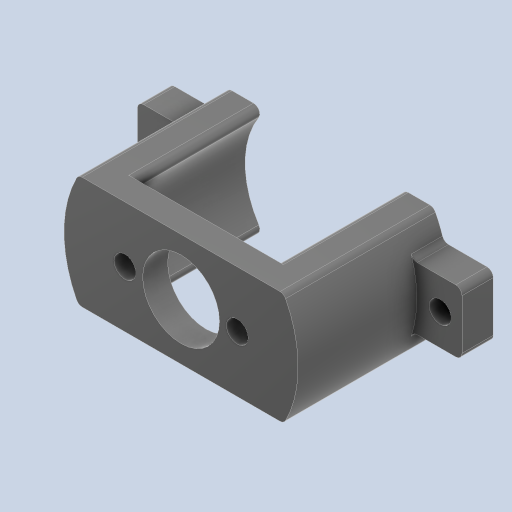
# Autodesk Inventor part: encoderholder
Saved by Autodesk Inventor 2024 (Build 280153000, 153)
## iProperties
Created: 2023-08-25
Part Number: encoderholder
Material: ABS プラスチック
Document SubType Name: Modeling
Designer: zegi
Density: 1.06 g/cm^3
Appearance: 滑らか - 黒
Author: zegi
Autodesk Inventor part; units mm, degrees
ref_plane "YZ Plane" through (0, 0, 0) normal (1, 0, 0) x (0, 1, 0)
ref_plane "XZ Plane" through (0, 0, 0) normal (0, 1, 0) x (-1, 0, 0)
ref_plane "XY Plane" through (0, 0, 0) normal (0, 0, 1) x (1, 0, 0)
sketch "スケッチ2" plane through (0, 0, 0) normal (0, 0, 1) x (1, 0, 0)
  circle A0 centre (0, 0) radius 6.15
  circle A1 centre (9, 0) radius 1.75
  line L0 (0, 9) -> (16.4488, 9)
  line L1 (16.4488, -9) -> (0, -9)
  line L2 (0, -9) -> (0, 9)
  line L3 (0, 0) -> (10.75, 0) construction
  circle A2 centre (0, 0) radius 18.75
  line L4 (0, 0) -> (18.75, 0) construction
  circle A3 centre (0, 0) radius 13.75
  line L5 (0, 0) -> (13.75, 0)
  point P0 (0, 6.15)
  point P1 (0, -6.15)
  point P2 (10.3953, 9)
  point P3 (10.3953, -9)
  dimension "d6" = 3.5
  dimension "d5" = 12.3
  dimension "d7" = 9
  dimension "d11" = 18
  dimension "d12" = 5
  dimension "d20" = 3
  constraints: 12 end point, 3 coincident, 3 point on circle, 2 centre point, 2 horizontal, 2 horizontal alignment, 1 midpoint, 1 parallel, 1 perpendicular, 1 point on line, 1 vertical, 5 other
  measures "d5" diameter of A0
  measures "d7" distance of point (0, 0) point (9, 0)
  measures "d11" distance of L1.end L0.start
  measures "d20" distance of L5.end L3.end
extrude "押し出し1" add sketch "スケッチ2" along normal blind 4 contours L5 A1 A3 L1 L2 A0 | A0 L2 L0 A3 L5 A1 | L0 A2 L1 A3 picked at (14.4338, 5.2266)
extrude "押し出し2" add sketch "スケッチ2" against normal blind 15 contours L0 A2 L1 A3 picked at (14.4338, 5.2266)
sketch "スケッチ3" plane through (0, 0, -15) normal (0, 0, -1) x (-1, 0, 0)
  line L0 (-16.4488, -9) -> (-10.3953, -9) projected
  arc A0 (-10.3953, 9) -> (-10.3953, -9) centre (0, 0) ccw projected
  line L1 (-10.3953, 9) -> (-16.4488, 9) projected
  arc A1 (-16.4488, 9) -> (-16.4488, -9) centre (0, 0) ccw projected
  line L2 (-26, -9) -> (-10.3953, -9)
  line L3 (-10.3953, -9) -> (-10.3953, 9)
  line L4 (-10.3953, 9) -> (-26, 9)
  line L5 (-26, 9) -> (-26, -9)
  line L6 (-26, 0) -> (-10.3953, 0) construction
  circle A2 centre (-22.5, 0) radius 1.75
  line L7 (-26, 5) -> (-10.3953, 5)
  line L8 (-10.3953, 5) -> (-10.3953, -5)
  line L9 (-10.3953, -5) -> (-26, -5)
  line L10 (-26, -5) -> (-26, 5)
  point P0 (-18.071, -5)
  point P1 (-18.071, 5)
  point P2 (-26, -5)
  dimension "d17" = 3.5
  dimension "d18" = 22.5
  dimension "d19" = 3.5
  dimension "d24" = 10
  constraints: 18 end point, 4 parallel, 3 point on line, 2 horizontal, 2 midpoint, 2 perpendicular, 1 centre point, 1 other
  measures "d17" diameter of A2
  measures "d18" distance of A2.centre point (0, 0)
  measures "d19" distance from line of L5 A2.centre
  measures "d24" distance of L7.end L8.end
extrude "押し出し3" add sketch "スケッチ3" along normal blind 5 contours A1 L9 A0 L0 | L9 L5 L7 A1 | A1 L7 A0 L9 | A1 L1 A0 L7
fillet "フィレット1" radius 1 10 edges at (10.3953, 9, -10) (10.3953, -9, -10) (16.4488, 9, -5.5) (16.4488, 9, -17.5) (16.4488, -9, -17.5) (16.4488, -9, -5.5) (26, 5, -17.5) (26, -5, -17.5) (18.071, 5, -17.5) (18.071, -5, -17.5)
mirror "ミラー1" about plane through (0, 9, 0) normal (-1, 0, 0)
